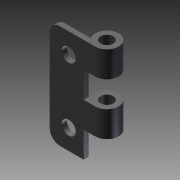
# Autodesk Inventor part: SHPSNA5_3
Saved by Autodesk Inventor 2011 SP1 (Build 150282100, 282)
## iProperties
Created: 2015-01-26
Part Number: SHPSNA5_3
Catalog Web Link: www.cadenas.de
Description: SHPSNA_3-Hinges with Slotted Holes
Vendor: MISUMI
Document SubType Name: Modeling
Designer: PARTuser1
Manufacturer: MISUMI
Mass: 2.02958 g
Surface Area: 23.6557 cm^2
Volume: 2.02958 cm^3
Density: 1 g/cm^3
Category: PARTsolutions
Company: MISUMI
Title: SHPSNA5_3
Author: Cadenas PARTsolutions
Comments: Hinges with Slotted Holes
PSOL_IDENT_0: {\\10.0.0.236\data_v8\23d-libs\misumi\metric\44_handles_hinges\shpsna_3.prj},162 {VTYP=3D},{NB=SHPSN
PSOL_IDENT_1: A5_3},{LINA=SHPSNA5_3},{NN=SHPSNA_3},{DATE=14.11.2014 09:15:25},{GEOMDATE=31.03.2009 09:27:00},{VERS
PSOL_IDENT_2: ION=},{LINEID=10},{LINESUBID=-1},{WBVAR=}  {NB=SHPSNA5_3},{LINA=SHPSNA5_3},{KT=DUMMY},{PN=SHPSNA5},{
PSOL_IDENT_3: TYPE=SHPSNA},{MAT=304 Stainless Steel},{NO=5},{AL1=9},{AL2=88},{MASS=43},{L=41},{W=36},{K=8},{P=25},
PSOL_IDENT_4: {J=7.5},{S=21},{N=5.5},{Z=5.5x6.5},{Z1=5.5},{Z2=6.5},{T=2},{E=4.6},{R=4.6},{CR=4},{D=5}
SUPPLIER: MISUMI
ARTICLENO: SHPSNA5_3
BOMINFO: SHPSNA5_3
CREATOR: CADENAS GmbH
Autodesk Inventor part; units mm, degrees
ref_plane "YZ Plane" through (0, 0, 0) normal (1, 0, 0) x (0, 1, 0)
ref_plane "XZ Plane" through (0, 0, 0) normal (0, 1, 0) x (-1, 0, 0)
ref_plane "XY Plane" through (0, 0, 0) normal (0, 0, 1) x (1, 0, 0)
sketch "Sketch_1" plane through (0, 0, 0) normal (0, 0, 1) x (1, 0, 0)
  line L0 (-18, -4.6) -> (0, -4.6)
  arc A0 (0, -4.6) -> (-3.7947, -2.6) centre (0, 0) ccw
  line L1 (-3.7947, -2.6) -> (-18, -2.6)
  line L2 (-18, -2.6) -> (-18, -4.6)
  circle A1 centre (0, 0) radius 2.5
  constraints: 6 end point, 2 centre point, 2 point on circle
extrude "Extrusion1" add sketch "Sketch_1" along normal blind 41
sketch "Sketch_2" plane through (0, -4.6, 0) normal (0, 1, 0) x (1, 0, 0)
  line L0 (-20, 2) -> (-20, -43)
  line L1 (-20, -43) -> (-9.2, -43)
  line L2 (-9.2, -43) -> (-9.2, -41)
  line L3 (-9.2, -41) -> (-14, -41)
  arc A0 (-18, -37) -> (-14, -41) centre (-14, -37) ccw
  line L4 (-18, -37) -> (-18, -4)
  arc A1 (-14, 0) -> (-18, -4) centre (-14, -4) ccw
  line L5 (-14, 0) -> (-9.2, 0)
  line L6 (-9.2, 0) -> (-9.2, 2)
  line L7 (-9.2, 2) -> (-20, 2)
  constraints: 16 end point, 4 point on circle, 2 centre point
extrude "Extrusion2" cut sketch "Sketch_2" along normal blind 2
sketch "Sketch_3" plane through (0, -4.6, 0) normal (0, 1, 0) x (1, 0, 0)
  circle A0 centre (-10.5, -33) radius 2.75
  constraints: 1 centre point
extrude "Extrusion3" cut sketch "Sketch_3" along normal blind 2
sketch "Sketch_4" plane through (0, -4.6, 0) normal (0, 1, 0) x (1, 0, 0)
  circle A0 centre (-10.5, -8) radius 2.75
  constraints: 1 centre point
extrude "Extrusion4" cut sketch "Sketch_4" along normal blind 2
sketch "Sketch_7" plane through (0, 0, 0) normal (0, 0, 1) x (1, 0, 0)
  line L0 (-4.6, -4.6) -> (0, -4.6)
  arc A0 (0, -4.6) -> (-4.6, 0) centre (0, 0) ccw
  line L1 (-4.6, 0) -> (-4.6, -4.6)
  constraints: 4 end point, 2 point on circle, 1 centre point
extrude "Extrusion5" cut sketch "Sketch_7" along normal blind 10.25
sketch "Sketch_5" plane through (0, 0, 30.75) normal (0, 0, 1) x (1, 0, 0)
  line L0 (-4.6, -4.6) -> (0, -4.6)
  arc A0 (0, -4.6) -> (-4.6, 0) centre (0, 0) ccw
  line L1 (-4.6, 0) -> (-4.6, -4.6)
  constraints: 4 end point, 2 point on circle, 1 centre point
extrude "Extrusion6" cut sketch "Sketch_5" against normal blind 10.25
ref_plane "3_to_1_XY" through (0, 0, 20.5) normal (0, 0, 1) x (1, 0, 0)
ref_plane "3_to_1_YZ" through (0, 0, 20.5) normal (1, 0, 0) x (0, 1, 0)
ref_plane "3_to_1_ZX" through (0, 0, 20.5) normal (0, 1, 0) x (0, 0, 1)
body "Solid1"
